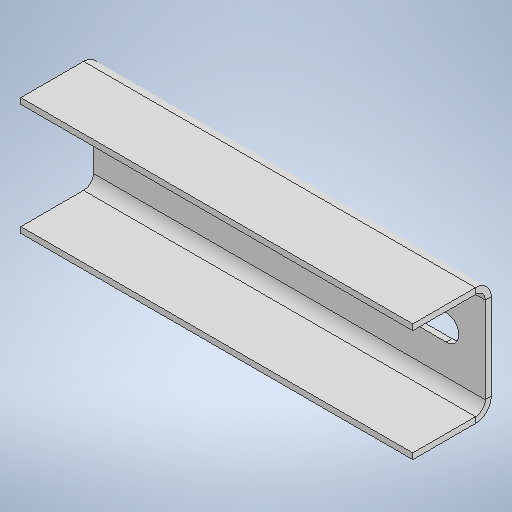
# Autodesk Inventor part: NDM-VOS 715 flange
Saved by Autodesk Inventor 2025 (Build 290162010, 162A)
## iProperties
Created: 2024-07-01
Part Number: NDM-VOS 715 flange
Material: Stainless Steel
Document SubType Name: Sheet Metal
Designer: user
Stock Number: МОО 902 опора рамы
Mass: 563.312 g
Surface Area: 499.957 cm^2
Volume: 70.414 cm^3
Density: 8 g/cm^3
Sheet Metal Rule: AISI304 3mm Die 32
Sheet Metal Width: 127,855 mm
Sheet Metal Length: 200,000 mm
Sheet Metal Area: 25570,973 mm^2
Appearance: Default
Flat Pattern Width: 12.7855 cm
Flat Pattern Length: 20 cm
Flat Pattern Area: 255.71 cm^2
Author: pokla
Autodesk Inventor part; units mm, degrees
ref_plane "YZ Plane" through (0, 0, 0) normal (1, 0, 0) x (0, 1, 0)
ref_plane "XZ Plane" through (0, 0, 0) normal (0, 1, 0) x (-1, 0, 0)
ref_plane "XY Plane" through (0, 0, 0) normal (0, 0, 1) x (1, 0, 0)
sketch "Sketch4" plane through (0, 0, 0) normal (0, 1, 0) x (-1, 0, 0)
  line L0 (100, -60) -> (-100, -60)
  line L1 (-100, -60) -> (-100, 0)
  line L2 (-100, 0) -> (100, 0)
  line L3 (100, 0) -> (100, -60)
  point P0 (0, 0)
  point P1 (0, 0)
  dimension "d36" = 200
  dimension "d37" = 60
  measures "d36" distance of L0.start L0.end
  measures "d37" distance between parallel lines of L0 L2
extrude "Plate2" add sketch "Sketch4" along normal blind 3
sketch "Sketch5" plane through (0, 0, 0) normal (0, -1, 0) x (1, 0, 0)
  circle A0 centre (-80, -30) radius 6.5
  circle A1 centre (80, -30) radius 6.5
  line L0 (0, 0) -> (0, -60) construction
  line L1 (100, -60) -> (-100, -60) construction
  line L2 (100, 0) -> (-100, 0) projected
  line L3 (80, -23.5) -> (-80, -23.5)
  line L4 (80, -36.5) -> (-80, -36.5)
  dimension "d39" = 160
  dimension "d40" = 30
  dimension "d41" = 13
  dimension "d55" = 60
  constraints: 6 end point, 4 point on circle, 4 tangent, 2 centre point, 1 midpoint, 1 other
  measures "d39" distance of A1.centre A0.centre
  measures "d40" distance from line of L1 A1.centre
  measures "d41" diameter of A1
  measures "d55" distance between parallel lines of L1 L2
extrude "Cut1" cut sketch "Sketch5" against normal blind 3
sketch "Sketch6" plane through (-100, 3, -3) normal (0, 0, 1) x (1, 0, 0)
  line L0 (200, 0) -> (0, 0)
  line L1 (0, 0) -> (0, -40)
  line L2 (0, -40) -> (200, -40)
  line L3 (200, -40) -> (200, 0)
  constraints: 6 end point, 1 horizontal, 1 perpendicular, 1 vertical
edge flange "Flange1" height 40 angle 90 thickness 3 bend radius 5 thickness toward (0, 0, 1) relief round relief width 3 relief depth 1.5 corner gap 5 corner form 0 edges at (0, 0, 0) (0, 0, -60) wall of the first edge with corners at (100, 3, -3) (-100, 3, -3) (-100, -37, -3) (100, -37, -3)
bend "Bend1"
corner "Corner1"
equation "\"d40\" = 0.5 * d55"
equation "\"d42\" = Thickness"
equation "\"d38\" = Thickness"
equation "\"d44\" = BendReliefWidth"
equation "\"d45\" = BendReliefDepth"
equation "\"d46\" = MinimumRemnant"
equation "\"d47\" = TransitionRadius"
equation "\"d50\" = BendRadius"
equation "\"d51\" = CornerReliefSize"
equation "\"d52\" = GapSize"
equation "\"d53\" = JacobiRadiusSize"
equation "\"BendReliefWidth\" = Thickness"
equation "\"BendReliefDepth\" = 0.5 * Thickness"
equation "\"CornerReliefSize\" = 4 * Thickness"
equation "\"MinimumRemnant\" = 2 * Thickness"
equation "\"TransitionRadius\" = BendRadius"
equation "\"JacobiRadiusSize\" = BendRadius"
equation "\"GapSize\" = Thickness"
equation "\"Thickness\" = 3"
equation "\"BendRadius\" = 5"
body "Solid2"
